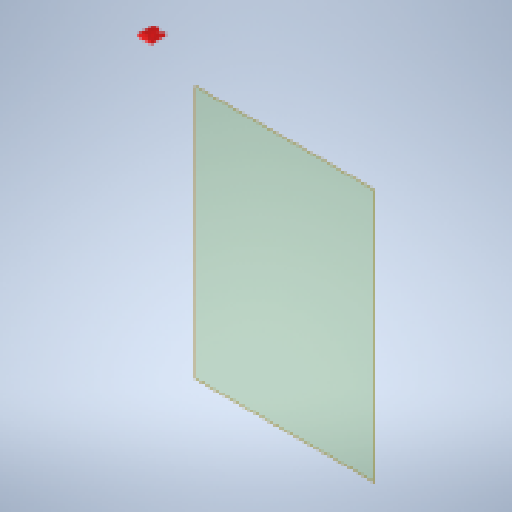
# Autodesk Inventor part: AxleHolder
Saved by Autodesk Inventor 2023 (Build 270158000, 158)
## iProperties
Created: 2023-08-18
Part Number: AxleHolder
Material: Generic
Document SubType Name: Modeling
Designer: Felix
Density: 1 g/cm^3
Appearance: Smooth - Red
Author: Felix
Autodesk Inventor part; units mm, degrees
ref_plane "YZ Plane" through (0, 0, 0) normal (1, 0, 0) x (0, 1, 0)
ref_plane "XZ Plane" through (0, 0, 0) normal (0, 1, 0) x (-1, 0, 0)
ref_plane "Work Plane2" through (234.4934, -62.0868, 206.5159) normal (0, 0, -1) x (-1, 0, 0)
sketch "Sketch3" plane through (234.4934, -62.0868, 206.5159) normal (0, 0, -1) x (-1, 0, 0)
  circle A0 centre (324.3, 410) radius 4 construction
  line L0 (314.485, 407) -> (320.2585, 417)
  line L1 (320.2585, 417) -> (328.3415, 417)
  line L2 (328.3415, 417) -> (334.115, 407)
  line L3 (-385, 402) -> (385, 402) construction
  line L4 (314.485, 407) -> (314.485, 402) construction
  line L5 (334.115, 407) -> (334.115, 402) construction
  line L6 (314.485, 407) -> (306.485, 407)
  line L7 (306.485, 407) -> (306.485, 402)
  line L8 (306.485, 402) -> (314.485, 402)
  line L9 (314.485, 402) -> (314.485, 407) construction
  line L10 (334.115, 407) -> (342.115, 407)
  line L11 (342.115, 407) -> (342.115, 402)
  line L12 (342.115, 402) -> (334.115, 402)
  line L13 (334.115, 402) -> (334.115, 407) construction
  line L14 (314.485, 402) -> (334.115, 402)
  point P0 (234.4934, 62.0868)
  dimension "d19" = 8
  dimension "d20" = 3
  dimension "d21" = 60
  dimension "d22" = 60
  dimension "d24" = 3
  dimension "d25" = 3
  dimension "d26" = 5
  dimension "d27" = 5
  dimension "d28" = 8
  dimension "d29" = 8
  constraints: 28 end point, 4 parallel, 4 perpendicular, 4 point on line, 3 horizontal, 1 centre point, 1 coincident, 1 collinear
  measures "d19" diameter of A0
  measures "d20" distance edge to line of A0 L1
  measures "d21" angle of L1 L0
  measures "d22" angle of L1 L2
  measures "d24" distance edge to line of A0 L0
  measures "d25" distance edge to line of A0 L2
  measures "d26" distance of L0.start L4.end
  measures "d27" distance of L2.end L5.end
  measures "d28" distance of L0.start L6.end
  measures "d29" distance of L2.end L10.end
ref_plane "Work Plane3" through (-75.5066, 299.1132, 245.5159) normal (0, 0, 1) x (1, 0, 0)
extrude "Extrusion2" add sketch "Sketch3" against normal up to surface (39 mm away)
sketch "Sketch4" plane through (234.4934, -62.0868, 206.5159) normal (0, 0, -1) x (-1, 0, 0)
  point P0 (234.4934, 62.0868)
  point P1 (324.3, 410)
hole "Hole2" at (-89.8066, 347.9132, 206.5159) direction (0, 0, 1) diameter 8.4 end through all counterbore diameter 18 counterbore depth 6.3 clearance for "Hex Head Cap Screw DIN EN 24017" size "M8" standard "DIN"
sketch "Sketch5" plane through (-79.9916, 344.9132, 206.5159) normal (0, 1, 0) x (1, 0, 0)
  line L0 (-119.515, -29) -> (748.485, -29) construction
  line L1 (-119.515, -9) -> (748.485, -9) construction
  line L2 (8, 0) -> (8, -39) construction
  line L3 (-27.6299, 0) -> (-27.6299, -39) construction
  point P0 (79.9916, 206.5159)
  point P1 (3, -29)
  point P2 (-22.6299, -29)
  point P3 (-22.6299, -9)
  point P4 (3, -9)
  dimension "d39" = 5
  dimension "d40" = 5
  dimension "d41" = 5
  dimension "d42" = 5
  constraints: 4 point on line
  measures "d39" distance from line of L2 point (3, -29)
  measures "d40" distance from line of L3 point (-22.63, -29)
  measures "d41" distance from line of L2 point (3, -9)
  measures "d42" distance from line of L3 point (-22.63, -9)
hole "Hole3" at (-76.9916, 344.9132, 235.5159) at (-102.6215, 344.9132, 235.5159) at (-102.6215, 344.9132, 215.5159) at (-76.9916, 344.9132, 215.5159) direction (0, -1, 0) diameter 4.3 end through all clearance for "Hex Head Cap Screw DIN EN 24017" size "M4" standard "DIN"
sketch "Sketch6" plane through (-79.9916, 344.9132, 206.5159) normal (0, 1, 0) x (1, 0, 0)
  point P0 (79.9916, 206.5159)
  point P1 (3, -29)
  point P2 (-22.6299, -29)
  point P3 (-22.6299, -9)
  point P4 (3, -9)
hole "Hole4" at (-76.9916, 344.9132, 235.5159) at (-102.6215, 344.9132, 235.5159) at (-102.6215, 344.9132, 215.5159) at (-76.9916, 344.9132, 215.5159) direction (0, 1, 0) diameter 11 end through all
sketch "Sketch7" plane through (234.4934, -62.0868, 206.5159) normal (0, 0, -1) x (-1, 0, 0)
  arc A0 (315.4094, 408.601) -> (320.1769, 402) centre (324.3, 410) ccw projected
  line L0 (315.4094, 408.601) -> (314.485, 407) projected
  line L1 (314.485, 407) -> (306.485, 407) projected
  line L2 (306.485, 407) -> (306.485, 402) projected
  line L3 (306.485, 402) -> (320.1769, 402) projected
  arc A1 (328.4231, 402) -> (333.1906, 408.601) centre (324.3, 410) ccw projected
  line L4 (328.4231, 402) -> (342.115, 402) projected
  line L5 (342.115, 402) -> (342.115, 407) projected
  line L6 (342.115, 407) -> (334.115, 407) projected
  line L7 (334.115, 407) -> (333.1906, 408.601) projected
  line L8 (320.2585, 417) -> (314.485, 407) projected
  line L9 (314.485, 407) -> (317.3718, 402)
  line L10 (306.485, 402) -> (342.115, 402) projected
  line L11 (342.115, 407) -> (334.115, 407) projected
  line L12 (334.115, 407) -> (331.2282, 402)
  point P0 (234.4934, 62.0868)
  point P1 (308.4231, 367)
  dimension "d63" = 60
  dimension "d64" = 60
  constraints: 4 end point, 2 point on line
  measures "d63" angle of L9 L1
  measures "d64" angle of L6 L12
extrude "Extrusion3" cut sketch "Sketch7" against normal up to surface (6.3 mm away) contours A0 L3 L9 L0 | A1 L7 L12 L4
equation "\"d22\" = d21"
equation "\"d24\" = d20"
equation "\"d25\" = d24"
equation "\"d27\" = d26"
equation "\"d29\" = d28"
equation "\"d40\" = d39"
equation "\"d41\" = d39"
equation "\"d42\" = d39"
body "Solid2"
